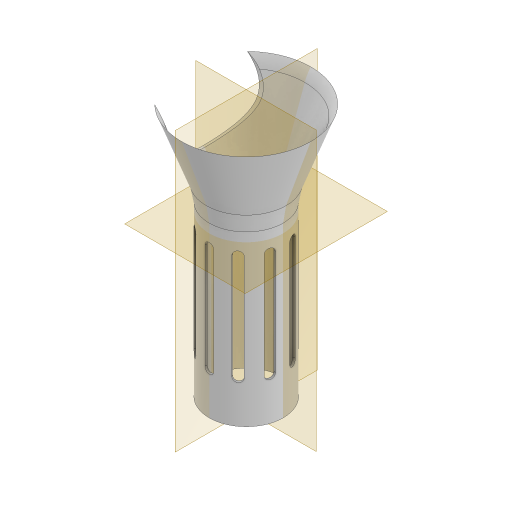
# Autodesk Inventor part: воронка
Saved by Autodesk Inventor 2023.2 (Build 272271030, 271C)
## iProperties
Created: 2025-04-19
Part Number: воронка
Material: Типовые
Document SubType Name: Modeling
Designer: Коноваленко
Density: 1 g/cm^3
Appearance: По умолчанию
Author: Коноваленко
Autodesk Inventor part; units mm, degrees
sketch "Эскиз1" plane through (0, 0, 0) normal (0, 0, 1) x (1, 0, 0)
  line L0 (0, 22.5937) -> (0, -11.0157) construction
  line L1 (49.4407, 74.3673) -> (27.5, 14.0856)
  line L2 (27.5, 14.0856) -> (27.5, -126.2141)
  line L3 (27.5, -126.2141) -> (29.2, -126.2141)
  line L4 (29.2, -126.2141) -> (29.2, 13.7859)
  line L5 (29.2, 13.7859) -> (51.0382, 73.7859)
  line L6 (51.0382, 73.7859) -> (49.4407, 74.3673)
  point P0 (0, 0)
  point P1 (38.4704, 44.2265)
  dimension "d0" = 1.7
  dimension "d1" = 1.7
  dimension "d3" = 27.5
  dimension "d7" = 140
  dimension "d23" = 160
  dimension "d24" = 60
  constraints: 15 end point, 3 perpendicular, 2 vertical, 1 midpoint, 1 parallel, 1 point on line
  measures "d0" distance between parallel lines of L4 L2
  measures "d1" distance from line of L5 point (38.47, 44.226)
  measures "d3" distance between parallel lines of L2 L0
  measures "d7" distance of L3.end L4.end
  measures "d23" angle of L4 L5
  measures "d24" vertical distance of L4.end L5.end
revolve "Вращение1" add sketch "Эскиз1" angle 360 about axis through (0, 22.5937, 0) along (0, -1, 0)
fillet "Сопряжение1" radius 26.5 1 edges at (-49.4407, 74.3673, 0)
sketch "Эскиз2" plane through (0, 0, 0) normal (0, 0, 1) x (1, 0, 0)
  line L0 (3.5, -96.2141) -> (-3.5, -96.2141)
  line L1 (-3.5, -96.2141) -> (-3.5, -6.2141)
  line L2 (-3.5, -6.2141) -> (3.5, -6.2141)
  line L3 (3.5, -6.2141) -> (3.5, -96.2141)
  line L4 (3.5, -96.2141) -> (-3.5, -6.2141) construction
  line L5 (-3.5, -96.2141) -> (3.5, -6.2141) construction
  line L6 (-27.5, -126.2141) -> (27.5, -126.2141) projected
  line L7 (0, 25.2428) -> (0, -151.4569) projected
  circle A0 centre (0, -9.7141) radius 3.5
  circle A1 centre (0, -92.7141) radius 3.5
  point P0 (0, 0)
  point P1 (0, -51.2141)
  point P2 (-3.5, -9.7141)
  point P3 (-3.5, -92.7141)
  point P4 (3.5, -92.7141)
  point P5 (3.5, -9.7141)
  dimension "d8" = 7
  dimension "d9" = 90
  dimension "d10" = 30
  constraints: 12 end point, 4 tangent, 3 point on line, 2 centre point, 2 midpoint, 2 parallel, 1 horizontal, 1 perpendicular
  measures "d8" distance of L1.end L2.end
  measures "d9" distance of L2.end L0.start
  measures "d10" distance between parallel lines of L6 L0
extrude "Выдавливание1" cut sketch "Эскиз2" along normal mid plane 67 contours A1 L7 | L7 A1 | A1 L7 A0 L3 | A1 L1 A0 L7 | A0 L7 | A0 L7
pattern_circular "Круговой массив2" count 10 over 360 about axis through (0, -56.0642, 0) along (0, -1, 0) of "Выдавливание1"
sketch "Эскиз3" plane through (0, 0, 0) normal (1, 0, 0) x (0, 1, 0)
  circle A0 centre (65.5919, 0) radius 37.5
  line L0 (-20.4959, 0) -> (122.9754, 0) projected
  line L1 (65.5919, 46.2467) -> (65.5919, -46.2467) projected
  point P0 (0, 0)
  dimension "d25" = 75
  constraints: 1 centre point, 1 midpoint, 1 point on line
  measures "d25" diameter of A0
extrude "Выдавливание2" cut sketch "Эскиз3" against normal up to next
chamfer "Фаска2" distance 6.75 angle 45 1 edges at (-29.2, 13.7859, 0)
